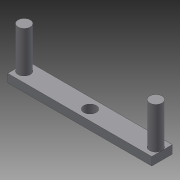
# Autodesk Inventor part: set color sensor
Saved by Autodesk Inventor 2015 (Build 190159000, 159)
## iProperties
Created: 2015-10-05
Part Number: set color sensor
Material: 一般
Document SubType Name: シート メタル
Designer: kenta
Density: 1 g/cm^3
Sheet Metal Rule: Default_mm
Appearance: 既定
Author: kenta
Autodesk Inventor part; units mm, degrees
ref_plane "YZ Plane" through (0, 0, 0) normal (1, 0, 0) x (0, 1, 0)
ref_plane "XZ Plane" through (0, 0, 0) normal (0, 1, 0) x (-1, 0, 0)
ref_plane "XY Plane" through (0, 0, 0) normal (0, 0, 1) x (1, 0, 0)
sketch "スケッチ1" plane through (0, 0, 0) normal (0, 0, 1) x (1, 0, 0)
  line L0 (-17.5, 2.5) -> (17.5, 2.5)
  line L1 (17.5, 2.5) -> (17.5, -2.5)
  line L2 (17.5, -2.5) -> (-17.5, -2.5)
  line L3 (-17.5, -2.5) -> (-17.5, 2.5)
  line L4 (-17.5, 2.5) -> (17.5, -2.5) construction
  line L5 (17.5, 2.5) -> (-17.5, -2.5) construction
  point P0 (0, 0)
  dimension "d0" = 5
  dimension "d1" = 35
  constraints: 12 end point, 2 midpoint, 2 parallel, 1 horizontal, 1 perpendicular
  measures "d0" distance of L0.end L1.end
  measures "d1" distance of L1.end L2.end
extrude "押し出し1" add sketch "スケッチ1" along normal blind 2
sketch "スケッチ2" plane through (0, 0, 2) normal (0, 0, 1) x (1, 0, 0)
  circle A0 centre (0, 0) radius 1.5
  dimension "d4" = 3
  constraints: 1 centre point, 1 coincident
  measures "d4" diameter of A0
extrude "押し出し2" cut sketch "スケッチ2" against normal blind 2
sketch "スケッチ3" plane through (0, 0, 2) normal (0, 0, 1) x (1, 0, 0)
  circle A0 centre (-16, 0) radius 1.5
  circle A1 centre (16, 0) radius 1.5
  circle A2 centre (0, 0) radius 1.5 projected
  dimension "d7" = 3
  dimension "d8" = 3
  dimension "d9" = 32
  dimension "d10" = 16
  dimension "d11" = 0
  constraints: 2 centre point
  measures "d7" diameter of A0
  measures "d8" diameter of A1
  measures "d9" distance of A1.centre A0.centre
  measures "d10" distance of A2.centre A0.centre
  measures "d11" vertical distance of A2.centre A0.centre
extrude "押し出し3" add sketch "スケッチ3" along normal blind 10 contours A0 | A1
equation "\"BendRadius\" = Thickness"
equation "\"BendReliefWidth\" = Thickness"
equation "\"BendReliefDepth\" = 0.5 * Thickness"
equation "\"CornerReliefSize\" = 4 * Thickness"
equation "\"MinimumRemnant\" = 2 * Thickness"
equation "\"TransitionRadius\" = BendRadius"
equation "\"JacobiRadiusSize\" = BendRadius"
equation "\"GapSize\" = Thickness"
equation "\"Thickness\" = 0.5"
